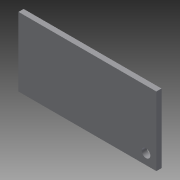
# Autodesk Inventor part: płaskownik
Saved by Autodesk Inventor 2014 (Build 180170000, 170)
## iProperties
Created: 2014-12-22
Part Number: płaskownik
Material: Ogólny
Document SubType Name: Modeling
Designer: Kuba
Density: 1 g/cm^3
Appearance: Domyślna
Author: Kuba
Autodesk Inventor part; units mm, degrees
ref_plane "YZ Plane" through (0, 0, 0) normal (1, 0, 0) x (0, 1, 0)
ref_plane "XZ Plane" through (0, 0, 0) normal (0, 1, 0) x (-1, 0, 0)
ref_plane "XY Plane" through (0, 0, 0) normal (0, 0, 1) x (1, 0, 0)
sketch "Szkic1" plane through (0, 0, 0) normal (0, 1, 0) x (-1, 0, 0)
  line L0 (40, -20) -> (-40, -20)
  line L1 (-40, -20) -> (-40, 20)
  line L2 (-40, 20) -> (40, 20)
  line L3 (40, 20) -> (40, -20)
  line L4 (40, -20) -> (-40, 20) construction
  line L5 (-40, -20) -> (40, 20) construction
  point P0 (0, 0)
  dimension "d0" = 80
  dimension "d1" = 40
  constraints: 12 end point, 2 midpoint, 2 parallel, 1 horizontal, 1 perpendicular
  measures "d0" distance of L1.end L2.end
  measures "d1" distance of L0.end L1.end
extrude "Wyciągnięcie proste1" add sketch "Szkic1" along normal blind 3
sketch "Szkic2" plane through (0, 3, 0) normal (0, 1, 0) x (1, 0, 0)
  line L0 (40, 20) -> (-40, 20) projected
  line L1 (34, 14) -> (34, -14)
  line L2 (-34, -14) -> (-34, 14)
  line L3 (-34, 14) -> (-6, 14)
  line L4 (-6, 14) -> (-6, -14)
  line L5 (-6, -14) -> (-34, -14)
  line L6 (-34, -14) -> (-34, 14)
  line L7 (34, 14) -> (6, 14)
  line L8 (6, 14) -> (6, -14)
  line L9 (6, -14) -> (34, -14)
  line L10 (34, -14) -> (34, 14)
  line L11 (6, 14) -> (34, -14) construction
  line L12 (34, 14) -> (6, -14) construction
  line L13 (-6, 14) -> (-34, -14) construction
  line L14 (-34, 14) -> (-6, -14) construction
  point P0 (0, 0)
  point P1 (-20, 0)
  point P2 (20, 0)
  dimension "d16" = 6
  dimension "d17" = 12
  constraints: 28 end point, 6 parallel, 5 perpendicular, 2 midpoint
  measures "d16" distance between parallel lines of L0 L3
  measures "d17" distance between parallel lines of L8 L4
hole "Otwór1" at (34, 3, -14) at (34, 3, 14) at (-34, 3, 14) at (-34, 3, -14) at (6, 3, 14) at (-6, 3, 14) at (6, 3, -14) at (-6, 3, -14) at (20, 3, 0) at (-20, 3, 0) direction (0, -1, 0) diameter 5 end through all
equation "\"d17\" = 2 * d16"
